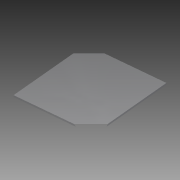
# Autodesk Inventor part: lid2
Saved by Autodesk Inventor 2015 (Build 190159000, 159)
## iProperties
Created: 2015-10-15
Part Number: lid2
Material: Polycarbonate, Clear
Description: insert part description/title
Document SubType Name: Modeling
Designer: c3132704
Density: 1.2 g/cm^3
Appearance: Polycarbonate - Clear
Part Category: insert part category here and press enter to fill value
Author: c3132704
Autodesk Inventor part; units mm, degrees
ref_plane "YZ Plane" through (0, 0, 0) normal (1, 0, 0) x (0, 1, 0)
ref_plane "XZ Plane" through (0, 0, 0) normal (0, 1, 0) x (-1, 0, 0)
ref_plane "XY Plane" through (0, 0, 0) normal (0, 0, 1) x (1, 0, 0)
sketch "Sketch1" plane through (0, 0, 0) normal (0, 0, 1) x (1, 0, 0)
  line L0 (-2.0956, 258.673) -> (-225.0857, 237.4269)
  line L1 (-225.0857, 237.4269) -> (-201.9426, -5.4731)
  line L2 (-201.9426, -5.4731) -> (21.0476, 15.773)
  line L3 (21.0476, 15.773) -> (-2.0956, 258.673)
  line L4 (18.7212, 19.1038) -> (-3.7511, 254.9628) construction
  line L5 (-7.2182, 256.1759) -> (-110.0796, 246.3754) construction
  line L6 (-87.3158, 7.4574) -> (15.5455, 17.2579) construction
  line L7 (-200.287, -1.763) -> (-222.7593, 234.0961) construction
  point P0 (0, 0)
  dimension "d6" = 2
  dimension "d7" = 2
  dimension "d8" = 2
  dimension "d9" = 2
  constraints: 8 end point, 4 parallel, 1 perpendicular
  measures "d6" distance between parallel lines of L4 L3
  measures "d7" distance between parallel lines of L6 L2
  measures "d8" distance between parallel lines of L7 L1
  measures "d9" distance between parallel lines of L5 L0
extrude "Extrusion1" add sketch "Sketch1" along normal blind 5
body "Solid1"
